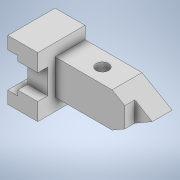
# Autodesk Inventor part: 2.3
Saved by Autodesk Inventor 2022 (Build 260153000, 153)
## iProperties
Created: 2023-04-17
Part Number: 2.3
Material: Genérico
Document SubType Name: Modeling
Designer: jpjoa
Density: 1 g/cm^3
Appearance: Padrão
Author: jpjoa
Autodesk Inventor part; units mm, degrees
ref_plane "YZ Plane" through (0, 0, 0) normal (1, 0, 0) x (0, 1, 0)
ref_plane "XZ Plane" through (0, 0, 0) normal (0, 1, 0) x (-1, 0, 0)
ref_plane "XY Plane" through (0, 0, 0) normal (0, 0, 1) x (1, 0, 0)
sketch "Esboço1" plane through (0, 0, 0) normal (0, 0, 1) x (1, 0, 0)
  line L0 (0, 0) -> (24, 0)
  line L1 (24, 0) -> (24, 10)
  line L2 (24, 10) -> (69.7513, 10)
  line L3 (69.7513, 10) -> (69.7513, 38)
  line L4 (69.7513, 38) -> (24, 38)
  line L5 (24, 38) -> (24, 48)
  line L6 (24, 48) -> (0, 48)
  line L7 (0, 48) -> (0, 38)
  line L8 (0, 38) -> (8, 38)
  line L9 (8, 38) -> (8, 34)
  line L10 (8, 34) -> (24, 34)
  line L11 (24, 34) -> (24, 14)
  line L12 (24, 14) -> (8, 14)
  line L13 (8, 14) -> (8, 10)
  line L14 (8, 10) -> (0, 10)
  line L15 (0, 10) -> (0, 0)
  line L16 (69.7513, 10) -> (94, 24)
  line L17 (94, 24) -> (69.7513, 38)
  line L18 (80, 32.0829) -> (80, 15.9171)
  line L19 (80, 32.0829) -> (96.1658, 32.0829) construction
  line L20 (8, 34) -> (8, 14)
  line L21 (24, 38) -> (24, 34)
  line L22 (24, 14) -> (24, 10)
  dimension "d13" = 24
  dimension "d14" = 60
  dimension "d15" = 28
  dimension "d16" = 94
  dimension "d17" = 8
  dimension "d18" = 16
  dimension "d19" = 48
  dimension "d20" = 28
  dimension "d21" = 20
  dimension "d22" = 90
  dimension "d23" = 14
  constraints: 46 end point, 14 perpendicular, 6 equal length, 5 point on line, 2 horizontal, 1 collinear
  measures "d13" distance of L0.start L0.end
  measures "d14" angle of L16 L17
  measures "d15" distance between parallel lines of L2 L4
  measures "d16" horizontal distance of L16.end L0.start
  measures "d17" distance of L7.end L8.end
  measures "d18" distance from line of L8.end L11
  measures "d19" distance of L0.start L6.end
  measures "d20" distance of L14.end L7.end
  measures "d21" distance of L12.end L9.end
  measures "d22" angle of L18 L19
  measures "d23" distance from line of L18 L16.end
extrude "Extrusão1" add sketch "Esboço1" along normal blind 38 contours L15 L14 L13 L12 L22 L1 L0 | L10 L9 L8 L7 L6 L5 L21
extrude "Extrusão2" add sketch "Esboço1" along normal blind 30 contours L12 L20 L10 L11
extrude "Extrusão3" add sketch "Esboço1" along normal blind 24 contours L22 L11 L21 L4 L3 L2 | L3 L17 L18 L16
extrude "Extrusão4" add sketch "Esboço1" along normal blind 16 contours L18 L17 L16
sketch "Esboço2" plane through (24, 10, 0) normal (0, -1, 0) x (1, 0, 0)
  circle A0 centre (26, 12) radius 5
  line L0 (0, 0) -> (45.7513, 0) projected
  line L1 (0, 0) -> (0, 38) projected
  point P0 (-24, 0)
  dimension "d32" = 10
  dimension "d33" = 12
  dimension "d34" = 26
  constraints: 1 centre point
  measures "d32" diameter of A0
  measures "d33" distance from line of L0 A0.centre
  measures "d34" distance from line of A0.centre L1
extrude "Extrusão5" cut sketch "Esboço2" against normal through all
